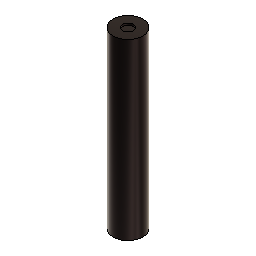
Inner Metal Cylinder v1 (Autodesk Fusion 360 design; units mm, degrees)
Autodesk Fusion 360 part; units mm, degrees
sketch "Sketch2" plane through (0, 0, 0) normal (0, 0, 1) x (1, 0, 0)
cylinder "CylinderPrimitive2" add diameter 137.3 height 804.8625 placed x (1, 0, 0) y (0, 1, 0) z (0, 0, 1) at (0, 0, 0)
sketch "Sketch3" plane through (0, 0, 804.8625) normal (0, 0, 1) x (-1, 0, 0)
  circle A0 centre (0, 0) radius 68.65
  circle A1 centre (0, 0) radius 25.25
  dimension "d5" = 50.5
  constraint coincident A0.centre A1.centre
  measures "d5" diameter of A1
extrude "Extrude1" cut sketch "Sketch3" against normal blind 28.575 contours A1
sketch "Sketch4" plane through (0, 0, 0) normal (0, 0, 1) x (1, 0, 0)
  circle A0 centre (0, 0) radius 25.25
  dimension "d8" = 50.5
  constraint coincident A0.centre origin
  measures "d8" diameter of A0
extrude "Extrude2" cut sketch "Sketch4" along normal blind 28.575
extrude "Extrude3" add 1 faces at (-8.0427, -2.4809, 776.2875) along direction (0, 0, 1) blind 28.575
extrude "Extrude4" add 1 faces at (4.2083, -8.3807, 28.575) along direction (0, 0, -1) blind 28.575
extrude "Extrude5" cut sketch "Sketch3" against normal blind 9.25 contours A1
extrude "Extrude6" cut sketch "Sketch4" along normal blind 9.25
equation "d3 = 31 11/16\""
